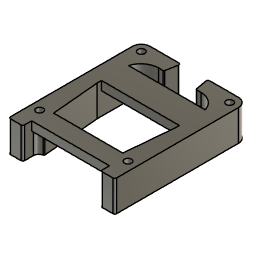
FlangeV3 v4 (Autodesk Fusion 360 design; units mm, degrees)
Autodesk Fusion 360 part; units mm, degrees
sketch "Sketch1" plane through (0, 0, 0) normal (0, 0, 1) x (1, 0, 0)
  line L0 (0, 0) -> (60, 0)
  line L1 (0, 0) -> (0, 25)
  line L2 (60, 0) -> (60, 25)
  line L3 (0, 25) -> (7, 25)
  line L4 (59, 25) -> (53, 25)
  line L5 (8, 67) -> (8, 81.82)
  line L6 (8, 26) -> (8, 31)
  line L7 (52, 67) -> (49.0457, 34.5028)
  line L8 (8, 67) -> (10.9543, 34.5028)
  line L9 (0, 25) -> (-10, 25)
  line L10 (1, 25) -> (8, 25)
  line L11 (52, 25) -> (60, 25)
  line L12 (52, 26) -> (52, 31)
  line L13 (52, 67) -> (52, 81.82)
  line L14 (20.95, 100) -> (39.05, 100)
  line L15 (5, 100) -> (20.95, 100)
  line L16 (39.05, 100) -> (55, 100)
  line L17 (20.5334, 91.82) -> (18, 91.82)
  line L18 (39.4666, 91.82) -> (42, 91.82)
  line L19 (20.95, 100) -> (21.25, 100)
  line L20 (39.05, 100) -> (38.75, 100)
  line L21 (22.2336, 98.8196) -> (21.0251, 92.2298)
  line L22 (37.7664, 98.8196) -> (38.9749, 92.2298)
  arc A0 (52, 81.82) -> (42, 91.82) centre (42, 81.82) ccw
  arc A1 (18, 91.82) -> (8, 81.82) centre (18, 81.82) ccw
  arc A2 (10.534, 33.9636) -> (8, 31) centre (11, 31) ccw
  arc A3 (52, 31) -> (49.466, 33.9636) centre (49, 31) ccw
  arc A4 (10.534, 33.9636) -> (10.9543, 34.5028) centre (10.4563, 34.4575) ccw
  arc A5 (49.0457, 34.5028) -> (49.466, 33.9636) centre (49.5437, 34.4575) ccw
  arc A6 (7, 25) -> (8, 26) centre (7, 26) ccw
  arc A7 (52, 26) -> (53, 25) centre (53, 26) ccw
  arc A8 (22.2336, 98.8196) -> (21.25, 100) centre (21.25, 99) ccw
  arc A9 (38.75, 100) -> (37.7664, 98.8196) centre (38.75, 99) ccw
  line L23 (0, 95) -> (0, 26)
  line L24 (60, 26) -> (60, 95)
  arc A10 (60, 95) -> (55, 100) centre (55, 95) ccw
  arc A11 (5, 100) -> (0, 95) centre (5, 95) ccw
  arc A12 (0, 26) -> (1, 25) centre (1, 26) ccw
  arc A13 (59, 25) -> (60, 26) centre (59, 26) ccw
  arc A14 (20.5334, 91.82) -> (21.0251, 92.2298) centre (20.5334, 92.32) ccw
  arc A15 (38.9749, 92.2298) -> (39.4666, 91.82) centre (39.4666, 92.32) ccw
  point P0 (22.45, 100)
  point P1 (37.55, 100)
  dimension "d1" = 60
  dimension "d2" = 25
  dimension "d3" = 25
  dimension "d4" = 8
  dimension "d5" = 8
  dimension "d12" = 42
  dimension "d16" = 44
  dimension "d20" = 10
  dimension "d27" = 1.5
  dimension "d28" = 1.5
  dimension "d29" = 10
  dimension "d30" = 10
  dimension "d31" = 3
  dimension "d32" = 3
  dimension "d33" = 0.5
  dimension "d34" = 0.5
  dimension "d35" = 1
  dimension "d36" = 1
  dimension "d37" = 1
  dimension "d38" = 1
  dimension "d39" = 5
  dimension "d40" = 5
  dimension "d41" = 1
  dimension "d42" = 1
  dimension "d43" = 0.5
  dimension "d44" = 0.5
  constraint coincident L0.start L1.start
  constraint horizontal L0
  constraint perpendicular L0 L1
  constraint perpendicular L0 L2
  constraint perpendicular L1 L3
  constraint coincident L11.start L10
  constraint perpendicular L3 L5
  constraint perpendicular L4 L12
  constraint perpendicular L1 L9
  constraint collinear L10 L11
  constraint collinear L12 L13
  constraint perpendicular L5 L17
  constraint perpendicular L13 L18
  constraint tangent L18 A0
  constraint tangent L13 A0
  constraint tangent L17 A1
  constraint tangent L5 A1
  constraint tangent L6 A2
  constraint tangent L12 A3
  constraint tangent L8 A4
  constraint tangent A2 A4
  constraint tangent L7 A5
  constraint tangent A3 A5
  constraint coincident L10.end L6
  constraint tangent L3 A6
  constraint tangent L6 A6
  constraint coincident L11.start L12
  constraint coincident L11.start L4
  constraint tangent L12 A7
  constraint tangent L4 A7
  constraint coincident P0 L19
  constraint coincident P0 L21
  constraint tangent L19 A8
  constraint tangent L21 A8
  constraint coincident P1 L20
  constraint coincident P1 L22
  constraint tangent L20 A9
  constraint tangent L22 A9
  constraint perpendicular L10 L23
  constraint perpendicular L16 L24
  constraint tangent L24 A10
  constraint tangent L16 A10
  constraint tangent L23 A11
  constraint tangent L15 A11
  constraint coincident L1.end L23
  constraint coincident L1.end L10
  constraint tangent L23 A12
  constraint tangent L10 A12
  constraint coincident L2.end L24
  constraint coincident L2.end L4
  constraint tangent L24 A13
  constraint tangent L4 A13
  constraint tangent L17 A14
  constraint tangent L21 A14
  constraint tangent L18 A15
  constraint tangent L22 A15
  measures "d1" distance of L0.start L0.end
  measures "d2" distance of L0.start L1.end
  measures "d3" distance of L0.end L2.end
  measures "d4" distance of L1.end L10.end
  measures "d5" distance of L2.end L11.start
  measures "d12" distance of L10.end L5.start
  measures "d16" distance of L5.start L7.start
  measures "d20" distance of L1.end L9.end
  measures "d27" distance of L14.start P0
  measures "d28" distance of L14.end P1
  measures "d29" radius of A0
  measures "d30" radius of A1
  measures "d31" radius of A2
  measures "d32" radius of A3
  measures "d33" radius of A4
  measures "d34" radius of A5
  measures "d35" radius of A6
  measures "d36" radius of A7
  measures "d37" radius of A8
  measures "d38" radius of A9
  measures "d39" radius of A10
  measures "d40" radius of A11
  measures "d41" radius of A12
  measures "d42" radius of A13
  measures "d43" radius of A14
  measures "d44" radius of A15
extrude "Extrude1" add sketch "Sketch1" along normal blind 15 contours L3 L5 L6 L8 L10 L14 L15 L17 L19 L21 A1 A2 A4 A6 A8 L23 A11 A12 A14 | L4 L7 L11 L12 L13 L14 L16 L18 L20 L22 A0 A3 A5 A7 A9 L24 A10 A13 A15 makes body 1 at (0, 72, 10) makes body 2 at (60, 49, 10)
sketch "Sketch3" plane through (0, 0, 15) normal (0, 0, 1) x (-1, 0, 0)
  line L0 (-55, -100) -> (-38.75, -100)
  arc A0 (-38.75, -100) -> (-37.7664, -98.8196) centre (-38.75, -99) ccw
  line L1 (-37.7664, -98.8196) -> (-38.9749, -92.2298)
  arc A1 (-38.9749, -92.2298) -> (-39.4666, -91.82) centre (-39.4666, -92.32) ccw
  line L2 (-39.4666, -91.82) -> (-42, -91.82)
  arc A2 (-52, -81.82) -> (-42, -91.82) centre (-42, -81.82) ccw
  line L3 (-52, -81.82) -> (-52, -67)
  line L4 (-52, -67) -> (-49.0457, -34.5028)
  arc A3 (-49.0457, -34.5028) -> (-49.466, -33.9636) centre (-49.5437, -34.4575) ccw
  arc A4 (-52, -31) -> (-49.466, -33.9636) centre (-49, -31) ccw
  line L5 (-52, -31) -> (-52, -26)
  arc A5 (-52, -26) -> (-53, -25) centre (-53, -26) ccw
  line L6 (-53, -25) -> (-59, -25)
  arc A6 (-59, -25) -> (-60, -26) centre (-59, -26) ccw
  line L7 (-60, -26) -> (-60, -95)
  arc A7 (-60, -95) -> (-55, -100) centre (-55, -95) ccw
  line L8 (-5, -100) -> (-5, -77)
  line L9 (-5, -77) -> (-5, -84.5)
  line L10 (-5, -84.5) -> (0, -84.5)
  line L11 (0, -84.5) -> (-60, -84.5)
  line L12 (-60, -84.5) -> (-60, -69.5)
  line L13 (-60, -69.5) -> (0, -69.5)
  line L14 (0, -69.5) -> (0, -84.5)
  line L15 (0, -40) -> (-60, -40)
  line L16 (-60, -40) -> (-60, -30)
  line L17 (-60, -30) -> (0, -30)
  line L18 (0, -30) -> (0, -40)
  dimension "d45" = 23
  dimension "d46" = 7.5
  dimension "d47" = 15
  constraint vertical L8
  constraint coincident L8 L9.end
  constraint perpendicular L8 L10
  constraint horizontal L11
  constraint vertical L12
  constraint horizontal L13
  constraint vertical L14
  constraint coincident L7 L12.end
  constraint horizontal L15
  constraint vertical L16
  constraint horizontal L17
  constraint vertical L18
  constraint coincident L7 L16.end
  measures "d45" distance of L8.start L8.end
  measures "d46" distance of L8.end L9.end
  measures "d47" distance of L10.end L13.end
extrude "Extrude3" add sketch "Sketch3" 1 faces at (2.6667, 62.6667, 15) along normal blind 5 on bodies 1 bodies 1 2
extrude "Extrude4" cut 2 faces at (2.6667, 62.6667, 0) (57.3333, 62.6667, 0) along direction (0, 0, 1) blind 2.5 on bodies 1 bodies 1
sketch "Sketch4" plane through (0, 0, 20) normal (0, 0, 1) x (-1, 0, 0)
  line L0 (0, -95) -> (0, -26)
  arc A0 (0, -26) -> (-1, -25) centre (-1, -26) ccw
  line L1 (-1, -25) -> (-7, -25)
  arc A1 (-7, -25) -> (-8, -26) centre (-7, -26) ccw
  line L2 (-8, -26) -> (-8, -30)
  line L3 (-8, -30) -> (-52, -30)
  line L4 (-52, -30) -> (-52, -26)
  arc A2 (-52, -26) -> (-53, -25) centre (-53, -26) ccw
  line L5 (-53, -25) -> (-59, -25)
  arc A3 (-59, -25) -> (-60, -26) centre (-59, -26) ccw
  line L6 (-60, -26) -> (-60, -95)
  arc A4 (-60, -95) -> (-55, -100) centre (-55, -95) ccw
  line L7 (-55, -100) -> (-38.75, -100)
  arc A5 (-38.75, -100) -> (-37.7664, -98.8196) centre (-38.75, -99) ccw
  line L8 (-37.7664, -98.8196) -> (-38.9749, -92.2298)
  arc A6 (-38.9749, -92.2298) -> (-39.4666, -91.82) centre (-39.4666, -92.32) ccw
  line L9 (-39.4666, -91.82) -> (-42, -91.82)
  arc A7 (-51.6342, -84.5) -> (-42, -91.82) centre (-42, -81.82) ccw
  line L10 (-51.6342, -84.5) -> (-8.3658, -84.5)
  arc A8 (-18, -91.82) -> (-8.3658, -84.5) centre (-18, -81.82) ccw
  line L11 (-18, -91.82) -> (-20.5334, -91.82)
  arc A9 (-20.5334, -91.82) -> (-21.0251, -92.2298) centre (-20.5334, -92.32) ccw
  line L12 (-21.0251, -92.2298) -> (-22.2336, -98.8196)
  arc A10 (-22.2336, -98.8196) -> (-21.25, -100) centre (-21.25, -99) ccw
  line L13 (-21.25, -100) -> (-5, -100)
  arc A11 (-5, -100) -> (0, -95) centre (-5, -95) ccw
  line L14 (-10.4545, -40) -> (-8, -67)
  line L15 (-8, -67) -> (-8, -69.5)
  line L16 (-8, -69.5) -> (-52, -69.5)
  line L17 (-52, -69.5) -> (-52, -67)
  line L18 (-52, -67) -> (-49.5455, -40)
  line L19 (-49.5455, -40) -> (-10.4545, -40)
  circle A12 centre (-5, -95) radius 2
  circle A13 centre (-55, -95) radius 2
  dimension "d52" = 4
  dimension "d53" = 4
  constraint concentric A11 A12
  constraint concentric A4 A13
  measures "d52" diameter of A12
  measures "d53" diameter of A13
sketch "Sketch5" plane through (0, 0, 2.5) normal (0, 0, -1) x (1, 0, 0)
  line L0 (20.5334, -91.82) -> (18, -91.82)
  arc A0 (8, -81.82) -> (18, -91.82) centre (18, -81.82) ccw
  line L1 (8, -81.82) -> (8, -67)
  line L2 (8, -67) -> (10.9543, -34.5028)
  arc A1 (10.9543, -34.5028) -> (10.534, -33.9636) centre (10.4563, -34.4575) ccw
  arc A2 (8, -31) -> (10.534, -33.9636) centre (11, -31) ccw
  line L3 (8, -31) -> (8, -26)
  arc A3 (8, -26) -> (7, -25) centre (7, -26) ccw
  line L4 (7, -25) -> (1, -25)
  arc A4 (1, -25) -> (0, -26) centre (1, -26) ccw
  line L5 (0, -26) -> (0, -95)
  arc A5 (0, -95) -> (5, -100) centre (5, -95) ccw
  line L6 (5, -100) -> (21.25, -100)
  arc A6 (21.25, -100) -> (22.2336, -98.8196) centre (21.25, -99) ccw
  line L7 (22.2336, -98.8196) -> (21.0251, -92.2298)
  arc A7 (21.0251, -92.2298) -> (20.5334, -91.82) centre (20.5334, -92.32) ccw
  line L8 (5, -95) -> (5, -37.5)
  circle A8 centre (5, -37.5) radius 2
  line L9 (55, -95) -> (55, -37.5)
  circle A9 centre (55, -37.5) radius 2
  dimension "d55" = 57.5
  dimension "d56" = 4
  dimension "d57" = 57.5
  dimension "d58" = 4
  constraint coincident A5.centre L8.start
  constraint parallel L5 L8
  constraint coincident L8.end A8.centre
  constraint vertical L9
  constraint coincident L9.end A9.centre
  measures "d55" distance of A5.centre L8.end
  measures "d56" diameter of A8
  measures "d57" distance of L9.start L9.end
  measures "d58" diameter of A9
extrude "Extrude5" cut sketch "Sketch4" against normal blind 17.5 contours A12 | A13 bodies 1
extrude "Extrude6" cut sketch "Sketch5" against normal blind 17.5 contours A8 | A9 bodies 1
sketch "Sketch2" plane through (0, 0, 15) normal (0, 0, 1) x (-1, 0, 0)
  line L0 (-52, -31) -> (-52, -26)
  line L1 (-52, -81.82) -> (-52, -67)
  line L2 (-52, -67) -> (-49.0457, -34.5028)
  line L3 (-55, -100) -> (10, -100)
  line L4 (10, -100) -> (10, -85)
  line L5 (10, -85) -> (-55, -85)
  line L6 (-55, -85) -> (-55, -100)
  line L7 (10, -25) -> (-70, -25)
  line L8 (-70, -25) -> (-70, -35)
  line L9 (-70, -35) -> (10, -35)
  line L10 (10, -35) -> (10, -25)
  line L11 (-55, -100) -> (-38.75, -100)
  line L12 (-37.7664, -98.8196) -> (-38.9749, -92.2298)
  line L13 (-39.4666, -91.82) -> (-42, -91.82)
  arc A0 (-38.75, -100) -> (-37.7664, -98.8196) centre (-38.75, -99) ccw
  arc A1 (-38.9749, -92.2298) -> (-39.4666, -91.82) centre (-39.4666, -92.32) ccw
  arc A2 (-52, -81.82) -> (-42, -91.82) centre (-42, -81.82) ccw
  arc A3 (-49.0457, -34.5028) -> (-49.466, -33.9636) centre (-49.5437, -34.4575) ccw
  arc A4 (-52, -31) -> (-49.466, -33.9636) centre (-49, -31) ccw
  arc A5 (-52, -26) -> (-53, -25) centre (-53, -26) ccw
  line L14 (-53, -25) -> (-59, -25)
  arc A6 (-59, -25) -> (-60, -26) centre (-59, -26) ccw
  line L15 (-60, -26) -> (-60, -95)
  arc A7 (-60, -95) -> (-55, -100) centre (-55, -95) ccw
  constraint horizontal L3
  constraint vertical L4
  constraint horizontal L5
  constraint vertical L6
  constraint coincident L3.start L6.end
  constraint horizontal L7
  constraint vertical L8
  constraint horizontal L9
  constraint vertical L10
extrude "Extrude2" [suppressed]
